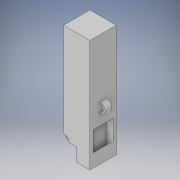
# Autodesk Inventor part: lower leg
Saved by Autodesk Inventor 2019 (Build 230136000, 136)
## iProperties
Created: 2018-07-06
Part Number: lower leg
Material: Generic
Document SubType Name: Modeling
Designer: HIVE
Density: 1 g/cm^3
Appearance: Default
Author: HIVE
Autodesk Inventor part; units mm, degrees
ref_plane "YZ Plane" through (0, 0, 0) normal (1, 0, 0) x (0, 1, 0)
ref_plane "XZ Plane" through (0, 0, 0) normal (0, 1, 0) x (-1, 0, 0)
ref_plane "XY Plane" through (0, 0, 0) normal (0, 0, 1) x (1, 0, 0)
sketch "Sketch1" plane through (0, 0, 0) normal (0, 1, 0) x (-1, 0, 0)
  line L0 (0, 0) -> (40, 0)
  line L1 (40, 0) -> (40, -40)
  line L2 (40, -40) -> (0, -40)
  line L3 (0, -40) -> (0, 0)
  dimension "d9" = 40
  dimension "d10" = 40
  constraints: 8 end point, 2 parallel, 1 horizontal, 1 perpendicular
  measures "d9" distance of L1.end L2.end
  measures "d10" distance of L0.end L1.end
extrude "Extrusion1" add sketch "Sketch1" along normal blind 150
ref_plane "Work Plane1" through (-40, 0, -20) normal (0, 0, 1) x (1, 0, 0)
sketch "Sketch2" plane through (-40, 0, -20) normal (0, 0, 1) x (1, 0, 0)
  line L0 (40, 0) -> (0, 0) projected
  line L1 (40, 0) -> (40, 150) projected
  line L2 (0, 150) -> (40, 150) projected
  line L3 (0, 0) -> (0, 150) projected
  line L4 (40, 0.2) -> (29.8, -10)
  line L5 (29.8, -10) -> (29.8, 40.6)
  line L6 (29.8, 40.6) -> (40, 30.4)
  line L7 (40, 0) -> (40, 150) projected
  arc A0 (40, 48.6) -> (40, 58.6) centre (40, 53.6) ccw
  arc A1 (40, 45.6) -> (40, 61.6) centre (40, 53.6) ccw
  circle A2 centre (0, 0) radius 5.1
  line L8 (0, 0) -> (40, 0) projected
  circle A3 centre (0, 0) radius 7.9
  line L9 (40, 0) -> (0, 0) projected
  circle A4 centre (0, 0) radius 8.1
  line L10 (40, 0) -> (20, 0)
  line L11 (20, 0) -> (20, -20)
  line L12 (20, -20) -> (40, -20)
  line L13 (40, -20) -> (40, 0)
  line L14 (40, 0.2) -> (40, 30.4)
  dimension "d2" = 45
  dimension "d3" = 45
  dimension "d5" = 10.2
  dimension "d8" = 30.2
  dimension "d12" = 5
  dimension "d13" = 8
  dimension "d14" = 5
  dimension "d17" = 10.2
  dimension "d18" = 15.8
  dimension "d27" = 16.2
  dimension "d28" = 20
  dimension "d29" = 10
  dimension "d30" = 10
  constraints: 16 end point, 7 point on line, 5 centre point, 4 point on circle, 3 coincident, 2 parallel, 1 collinear, 1 horizontal, 1 perpendicular, 1 vertical
  measures "d2" angle of L1 L6
  measures "d3" angle of L1 L4
  measures "d5" distance between parallel lines of L1 L5
  measures "d8" distance of L4.start L6.end
  measures "d12" vertical distance of L5.end A1.start
  measures "d13" radius of A1
  measures "d14" radius of A0
  measures "d17" diameter of A2
  measures "d18" diameter of A3
  measures "d27" diameter of A4
  measures "d28" distance of L12.end L11.end
  measures "d29" distance from line of L10 L4.end
  measures "d30" distance from line of L12 L4.end
extrude "Extrusion3" add sketch "Sketch2" along normal mid plane 10 contours L1 A0 A1
extrude "Extrusion4" add sketch "Sketch2" along normal mid plane 19.6 contours A3 L3 A2 L0 | L0 A2 L3 A3
extrude "Extrusion5" cut sketch "Sketch2" along normal through all both and the other way through all contours A2 L3 L0 | L0 L3 A2
extrude "Extrusion6" cut sketch "Sketch2" along normal up to surface (10.2 mm away) from surface at 9.8 contours A4 L3 A3 L0 | L0 A3 L3 A4 | A3 L3 A2 L0 | L0 A2 L3 A3
extrude "Extrusion7" cut sketch "Sketch2" against normal up to surface (10.2 mm away) from surface at -9.8 contours A4 L3 A3 L0 | L0 A3 L3 A4 | A3 L3 A2 L0 | L0 A2 L3 A3
extrude "Extrusion9" add sketch "Sketch2" along normal mid plane 40 contours L0 L5 L4 L13 L12 L11 | L0 L4 L5
extrude "Extrusion8" cut sketch "Sketch2" along normal mid plane 30.2 contours L5 L6 L1 L4 L0 | L0 L4 L5
equation "\"d9\" = legDiam"
equation "\"d10\" = legDiam"
equation "\"d5\" = kneeBallBaseH + clearance"
equation "\"d8\" = kneeBallBaseW + clearance"
equation "\"d17\" = hingeHoleDiam + clearance"
equation "\"d28\" = kneeBallDepth"
equation "\"d29\" = kneeBallLocationUp"
equation "\"d30\" = kneeBallLocationExtend"
equation "\"d19\" = 0.5 * legDiam - 2 * clearance"
equation "\"d33\" = legDiam"
equation "\"d31\" = kneeBallBaseW + clearance"
equation "\"legDiam\" = 40"
equation "\"kneeBallBaseH\" = 10"
equation "\"clearance\" = 0.2"
equation "\"kneeBallBaseW\" = 30"
equation "\"hingeHoleDiam\" = 10"
equation "\"kneeBallDepth\" = 20"
equation "\"kneeBallLocationUp\" = 10"
equation "\"kneeBallLocationExtend\" = 10"
body "Solid1"
